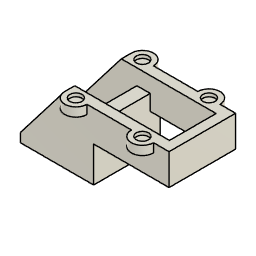
colour_sensor_holder (Autodesk Fusion 360 design; units mm, degrees)
part number: 2025-08-24-10-22-08-973
Autodesk Fusion 360 part; units mm, degrees
sketch "Base" plane through (0, 0, 0) normal (0, 0, 1) x (1, 0, 0)
  line L0 (0, 0) -> (33, 0)
  line L1 (33, 0) -> (33, 30)
  line L2 (33, 30) -> (0, 30)
  line L3 (0, 30) -> (0, 0)
  dimension "d2" = 33
  dimension "d3" = 30
  constraint horizontal L0
  constraint vertical L1
  constraint horizontal L2
  constraint vertical L3
  constraint coincident L0.start L3.end
  measures "d2" distance of L0.start L0.end
  measures "d3" distance of L0.end L1.end
extrude "Extrude1" add sketch "Base" along normal blind 4
sketch "Side Profile" plane through (0, 0, 0) normal (0, -1, 0) x (1, 0, 0)
  line L0 (0, 0) -> (33, 0)
  line L1 (33, 0) -> (33, 4)
  line L2 (33, 4) -> (0, 4)
  line L3 (0, 4) -> (0, 0)
  line L4 (33, 4) -> (33, 16)
  line L5 (33, 16) -> (67, 16)
  line L6 (67, 16) -> (67, 30)
  line L7 (67, 30) -> (20, 30)
  line L8 (20, 30) -> (0, 4)
  dimension "d6" = 12
  dimension "d7" = 34
  dimension "d8" = 14
  dimension "d9" = 47
  dimension "d10" = 52.431
  dimension "d11" = 33
  constraint coincident L1.end L2.start
  constraint perpendicular L2 L4
  constraint perpendicular L4 L5
  constraint perpendicular L5 L6
  constraint perpendicular L6 L7
  constraint coincident L2.end L3.start
  measures "d6" distance of L1.end L4.end
  measures "d7" distance of L4.end L5.end
  measures "d8" distance of L5.end L6.end
  measures "d9" distance of L6.end L7.end
  measures "d10" angle of L2 L8
  measures "d11" distance of L0.start L0.end
extrude "Extrude2" add sketch "Side Profile" against normal blind 4.5 contours L2 L4 L5 L6 L7 L8
extrude "Extrude3" add sketch "Side Profile" against normal blind 4.5 from surface at -25.5 contours L2 L4 L5 L6 L7 L8
sketch "Front End" plane through (0, 0, 0) normal (0, -1, 0) x (1, 0, 0)
  line L0 (0, 0) -> (33, 0)
  line L1 (33, 0) -> (33, 16)
  line L2 (33, 16) -> (67, 16)
  line L3 (67, 16) -> (67, 30)
  line L4 (67, 30) -> (20, 30)
  line L5 (20, 30) -> (0, 4)
  line L6 (0, 4) -> (0, 0)
  line L7 (67, 30) -> (62.7, 30)
  line L8 (62.7, 30) -> (62.7, 16)
  line L9 (62.7, 16) -> (67, 16)
  line L10 (67, 16) -> (67, 30)
  dimension "d17" = 4.3
  constraint horizontal L7
  constraint vertical L8
  constraint horizontal L9
  constraint vertical L10
  constraint coincident L3.end L4.start
  constraint collinear L2 L9
  measures "d17" distance of L3.end L7.end
extrude "Extrude4" add sketch "Front End" against normal blind 30 contours L2 L3 L4 L7 L8 L9 L10
sketch "Middle End" plane through (0, 0, 0) normal (0, -1, 0) x (1, 0, 0)
  line L0 (67, 30) -> (20, 30)
  line L1 (20, 30) -> (0, 4)
  line L2 (0, 4) -> (0, 0)
  line L3 (0, 0) -> (33, 0)
  line L4 (33, 0) -> (33, 16)
  line L5 (33, 16) -> (67, 16)
  line L6 (67, 16) -> (67, 30)
  line L7 (33, 23) -> (27, 23)
  line L8 (27, 23) -> (27, 0)
  line L9 (27, 0) -> (33, 0)
  line L10 (33, 0) -> (33, 23)
  dimension "d20" = 7
  dimension "d21" = 6
  constraint horizontal L7
  constraint vertical L8
  constraint horizontal L9
  constraint vertical L10
  constraint collinear L4 L10
  constraint collinear L3 L9
  measures "d20" distance of L0 L7
  measures "d21" distance of L7.start L7.end
extrude "Extrude5" add sketch "Middle End" against normal blind 30 contours L3 L4 L7 L8 L9 L10
sketch "Lip" plane through (62.7, 0, 0) normal (-1, 0, 0) x (0, -1, 0)
  line L0 (-25.5, 30) -> (-25.5, 16)
  line L1 (-25.5, 16) -> (-4.5, 16)
  line L2 (-4.5, 16) -> (-4.5, 30)
  line L3 (-4.5, 30) -> (-25.5, 30)
  line L4 (-18, 25) -> (-12, 25)
  line L5 (-12, 25) -> (-12, 21)
  line L6 (-12, 21) -> (-18, 21)
  line L7 (-18, 21) -> (-18, 25)
  dimension "d24" = 5
  dimension "d25" = 6
  dimension "d26" = 4
  dimension "d27" = 7.5
  constraint horizontal L4
  constraint vertical L5
  constraint horizontal L6
  constraint vertical L7
  measures "d24" distance of L3 L4
  measures "d25" distance of L4.start L4.end
  measures "d26" distance of L4.start L6.end
  measures "d27" distance of L0 L7
extrude "Extrude6" add sketch "Lip" along normal blind 4 contours L4 L5 L6 L7
sketch "Magnet Holders" plane through (0, 0, 30) normal (0, 0, 1) x (-1, 0, 0)
  line L0 (-67, -30) -> (-20, -30)
  line L1 (-20, -30) -> (-20, -25.5)
  line L2 (-20, -25.5) -> (-62.7, -25.5)
  line L3 (-62.7, -25.5) -> (-62.7, -4.5)
  line L4 (-62.7, -4.5) -> (-20, -4.5)
  line L5 (-20, -4.5) -> (-20, 0)
  line L6 (-20, 0) -> (-67, 0)
  line L7 (-67, 0) -> (-67, -30)
  circle A0 centre (-55, -30) radius 5
  circle A1 centre (-25, -30) radius 5
  circle A2 centre (-25, 0) radius 5
  circle A3 centre (-55, 0) radius 5
  circle A4 centre (-25, 0) radius 2.75
  circle A5 centre (-55, 0) radius 2.75
  circle A6 centre (-25, -30) radius 2.75
  circle A7 centre (-55, -30) radius 2.75
  dimension "d33" = 10
  dimension "d34" = 10
  dimension "d35" = 10
  dimension "d36" = 10
  dimension "d37" = 12
  dimension "d38" = 12
  dimension "d39" = 5
  dimension "d40" = 5
  dimension "d43" = 5.5
  dimension "d44" = 5.5
  dimension "d45" = 5.5
  dimension "d46" = 5.5
  constraint coincident L0 A0.centre
  constraint coincident L0 A1.centre
  constraint coincident L6 A2.centre
  constraint coincident L6 A3.centre
  constraint concentric A2 A4
  constraint concentric A3 A5
  constraint concentric A1 A6
  constraint concentric A0 A7
  measures "d33" diameter of A0
  measures "d34" diameter of A1
  measures "d35" diameter of A2
  measures "d36" diameter of A3
  measures "d37" distance of L6.end A3.centre
  measures "d38" distance of L0.start A0.centre
  measures "d39" distance of L0.end A1.centre
  measures "d40" distance of L5.end A2.centre
  measures "d43" diameter of A4
  measures "d44" diameter of A5
  measures "d45" diameter of A6
  measures "d46" diameter of A7
extrude "Extrude8" add sketch "Magnet Holders" against normal blind 4 contours L0 A7 | L0 A0 A7 | L0 A1 A6 | L0 A6 | L6 A3 A5 | L6 A5 | L6 A2 A4 | L6 A4 picked at (-54.1334, -30.6679) picked at (-25.1937, -31.0303) picked at (-55.7025, 1.0303) picked at (-24.1138, 0.4068)
extrude "Extrude9" cut sketch "Magnet Holders" against normal blind 1.5 contours L0 A7 | L0 A7 | L0 A6 | L0 A6 | L6 A5 | L6 A5 | L6 A4 | L6 A4
equation "base_plate_thickness = 4 mm" comment "Thickness of the Colour Detection Mechanism Platform's base plate."
equation "d4 = base_plate_thickness"
equation "d37 = 7 mm + 5 mm"
equation "d38 = 7 mm + 5 mm"
named bodies: "Colour Sensor Holder"
